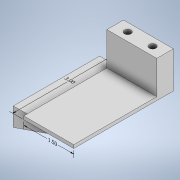
# Autodesk Inventor part: Base
Saved by Autodesk Inventor 2020 (Build 240168000, 168)
## iProperties
Created: 2020-02-17
Part Number: Base
Material: Generic
Document SubType Name: Modeling
Designer: maple
Density: 1 g/cm^3
Appearance: Default
Author: maple
Autodesk Inventor part; units mm, degrees
ref_plane "YZ Plane" through (0, 0, 0) normal (1, 0, 0) x (0, 1, 0)
ref_plane "XZ Plane" through (0, 0, 0) normal (0, 1, 0) x (-1, 0, 0)
ref_plane "XY Plane" through (0, 0, 0) normal (0, 0, 1) x (1, 0, 0)
sketch "Sketch1" plane through (0, 0, 0) normal (0, 1, 0) x (-1, 0, 0)
  line L0 (0, 0) -> (-38.1, 0)
  line L1 (-38.1, 0) -> (-38.1, -76.2)
  line L2 (-38.1, -76.2) -> (0, -76.2)
  line L3 (0, -76.2) -> (0, 0)
  dimension "d0" = 38.1
  dimension "d1" = 76.2
  constraints: 8 end point, 2 parallel, 1 horizontal, 1 perpendicular
  measures "d0" distance of L2.end L1.end
  measures "d1" distance of L1.end L0.end
extrude "Extrusion1" add sketch "Sketch1" along normal blind 2.54
sketch "Sketch2" plane through (0, 2.54, 0) normal (0, 1, 0) x (1, 0, 0)
  line L0 (38.1, 76.2) -> (0, 76.2) projected
  line L1 (0, 76.2) -> (38.1, 76.2)
  line L2 (38.1, 76.2) -> (38.1, 63.5)
  line L3 (38.1, 63.5) -> (0, 63.5)
  line L4 (0, 63.5) -> (0, 76.2)
  point P0 (0, 0)
  dimension "d4" = 38.1
  dimension "d5" = 12.7
  constraints: 8 end point, 2 parallel, 1 horizontal, 1 perpendicular
  measures "d4" distance of L2.end L3.end
  measures "d5" distance of L1.end L2.end
extrude "Extrusion2" add sketch "Sketch2" along normal blind 25.4
sketch "Sketch6" plane through (0, 27.94, 0) normal (0, 1, 0) x (1, 0, 0)
  line L0 (0, 76.2) -> (0, 63.5) projected
  line L1 (0, 69.85) -> (38.1, 69.85)
  line L2 (38.1, 63.5) -> (38.1, 76.2) projected
  line L3 (0, 69.85) -> (9.525, 69.85)
  line L4 (38.1, 69.85) -> (28.575, 69.85)
  point P0 (0, 0)
  dimension "d8" = 9.525
  dimension "d9" = 9.525
  constraints: 6 end point, 2 midpoint, 2 point on line
  measures "d8" distance of L1.start L3.end
  measures "d9" distance of L1.end L4.end
hole "Hole1" at (9.525, 27.94, -69.85) at (28.575, 27.94, -69.85) direction (0, -1, 0) diameter 5.08 depth 12.7 tip angle 118
sketch "Sketch7" plane through (0, 0, 0) normal (0, -1, 0) x (1, 0, 0)
  line L0 (38.1, 0) -> (38.1, -76.2) projected
  line L1 (38.1, -38.1) -> (27.94, -38.1)
  line L2 (38.1, -76.2) -> (0, -76.2) projected
  line L3 (19.05, -76.2) -> (19.05, -71.12)
  line L4 (0, 0) -> (38.1, 0) projected
  line L5 (19.05, 0) -> (19.05, -5.08)
  line L6 (19.05, -71.12) -> (38.1, -71.12)
  line L7 (27.94, -38.1) -> (27.94, -71.12)
  line L8 (27.94, -71.12) -> (-13.208, -71.12)
  line L9 (-13.208, -71.12) -> (-13.208, -5.08)
  line L10 (-13.208, -5.08) -> (27.94, -5.08)
  line L11 (27.94, -5.08) -> (27.94, -71.12)
  dimension "d23" = 10.16
  dimension "d24" = 5.08
  dimension "d25" = 5.08
  dimension "d26" = 41.148
  constraints: 18 end point, 3 midpoint, 3 perpendicular, 2 horizontal, 2 parallel, 2 point on line, 2 vertical
  measures "d23" distance of L1.start L1.end
  measures "d24" distance of L3.start L3.end
  measures "d25" distance of L5.start L5.end
  measures "d26" distance of L9.end L10.end
extrude "Extrusion3" add sketch "Sketch7" along normal blind 14.224 contours L7 L6 L8 L9 L10 L11
chamfer "Chamfer3" distance 41.148 distance2 14.224 1 edges at (27.94, -14.224, -38.1) measured on face at (14.224, -14.224, -49.1067)
body "Solid1"
